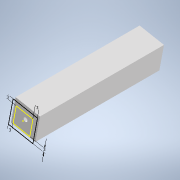
# Autodesk Inventor part: Casing
Saved by Autodesk Inventor 2021 (Build 250183000, 183)
## iProperties
Created: 2021-08-04
Part Number: Casing
Material: Generic
Document SubType Name: Modeling
Designer: techv
Density: 1 g/cm^3
Appearance: Default
Author: techv
Autodesk Inventor part; units mm, degrees
ref_plane "YZ Plane" through (0, 0, 0) normal (1, 0, 0) x (0, 1, 0)
ref_plane "XZ Plane" through (0, 0, 0) normal (0, 1, 0) x (-1, 0, 0)
ref_plane "XY Plane" through (0, 0, 0) normal (0, 0, 1) x (1, 0, 0)
sketch "Sketch1" plane through (0, 0, 0) normal (0, 0, 1) x (1, 0, 0)
  line L0 (7.598, 5.174) -> (-5.174, 7.598) projected
  line L1 (5.174, -7.598) -> (7.598, 5.174) projected
  line L2 (-7.598, -5.174) -> (5.174, -7.598) projected
  line L3 (-5.174, 7.598) -> (-7.598, -5.174) projected
  line L4 (-11.1048, -7.562) -> (-7.562, 11.1048)
  line L5 (-7.562, 11.1048) -> (11.1048, 7.562)
  line L6 (11.1048, 7.562) -> (7.562, -11.1048)
  line L7 (7.562, -11.1048) -> (-11.1048, -7.562)
  point P0 (0, 0)
  dimension "d0" = 3
  dimension "d1" = 3
  dimension "d2" = 3
  dimension "d3" = 3
  constraints: 8 end point, 4 parallel, 2 perpendicular
  measures "d0" distance between parallel lines of L0 L5
  measures "d1" distance between parallel lines of L3 L4
  measures "d2" distance between parallel lines of L7 L2
  measures "d3" distance between parallel lines of L6 L1
ref_plane "Work Plane1" through (0, 0, -5) normal (0, 0, 1) x (1, 0, 0)
sketch "Sketch2" plane through (0, 0, -5) normal (0, 0, 1) x (1, 0, 0)
  line L0 (7.598, 5.174) -> (-5.174, 7.598) projected
  line L1 (-7.562, 11.1048) -> (11.1048, 7.562) projected
  line L2 (-11.1048, -7.562) -> (-7.562, 11.1048) projected
  line L3 (7.562, -11.1048) -> (-11.1048, -7.562) projected
  line L4 (11.1048, 7.562) -> (7.562, -11.1048) projected
  line L5 (5.174, -7.598) -> (7.598, 5.174) projected
  line L6 (-7.598, -5.174) -> (5.174, -7.598) projected
  line L7 (-5.174, 7.598) -> (-7.598, -5.174) projected
  point P0 (0, 0)
extrude "Extrusion1" add sketch "Sketch2" against normal blind 92
sketch "Sketch3" plane through (0, 0, -5) normal (0, 0, 1) x (1, 0, 0)
  line L0 (-11.1048, -7.562) -> (7.562, -11.1048) projected
  line L1 (7.562, -11.1048) -> (11.1048, 7.562) projected
  line L2 (11.1048, 7.562) -> (-7.562, 11.1048) projected
  line L3 (-7.562, 11.1048) -> (-11.1048, -7.562) projected
  line L4 (7.598, 5.174) -> (5.174, -7.598) projected
  line L5 (5.174, -7.598) -> (-7.598, -5.174) projected
  line L6 (-7.598, -5.174) -> (-5.174, 7.598) projected
  line L7 (-5.174, 7.598) -> (7.598, 5.174) projected
  circle A0 centre (0, 0) radius 1.5
  dimension "d6" = 3
  constraints: 1 centre point, 1 coincident
  measures "d6" diameter of A0
extrude "Extrusion2" add sketch "Sketch3" along normal blind 3 contours L3 L2 L1 L0 | L4 L5 L6 L7
body "Solid1"
